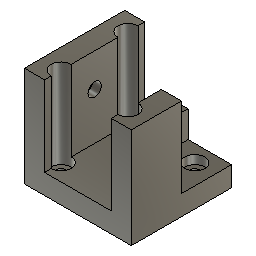
halter rakel neu v3 (Autodesk Fusion 360 design; units mm, degrees)
Autodesk Fusion 360 part; units mm, degrees
note: some values were not read from the file. Chosen so that the rebuilt part matches the saved one: which bodies a step acts on.
sketch "Skizze1" plane through (0, 0, 0) normal (0, 0, 1) x (1, 0, 0)
  line L0 (0, 0) -> (30, 0)
  line L1 (30, 0) -> (30, 30)
  line L2 (30, 30) -> (0, 30)
  line L3 (0, 30) -> (0, 0)
  line L4 (5, 25) -> (25, 25)
  line L5 (25, 25) -> (25, 5)
  line L6 (25, 5) -> (5, 5)
  line L7 (5, 5) -> (5, 25)
  circle A0 centre (5, 25) radius 1.5
  circle A1 centre (25, 25) radius 1.5
  circle A2 centre (5, 5) radius 1.5
  circle A3 centre (25, 5) radius 1.5
  dimension "d1" = 3
  dimension "d2" = 3
  dimension "d3" = 3
  dimension "d4" = 3
  constraint horizontal L0
  constraint vertical L1
  constraint horizontal L2
  constraint vertical L3
  constraint coincident L0.start L3.end
  constraint horizontal L4
  constraint vertical L5
  constraint horizontal L6
  constraint vertical L7
  constraint coincident L4.start L7.end
  constraint coincident L4.end L5.start
  constraint coincident L6.end L7.start
  constraint coincident L5.end L6.start
  measures "d1" diameter of A0
  measures "d2" diameter of A1
  measures "d3" diameter of A2
  measures "d4" diameter of A3
extrude "Extrusion1" add sketch "Skizze1" along normal blind 6 contours L0 L1 L2 L3 | L4 L5 L6 L7 A0 A1 A2 A3 makes body 1
sketch "Skizze2" plane through (0, 0, 6) normal (0, 0, 1) x (-1, 0, 0)
  circle A0 centre (-25, -5) radius 1.5
  circle A1 centre (-25, -25) radius 1.5
  circle A2 centre (-5, -5) radius 1.5
  circle A3 centre (-5, -25) radius 1.5
  line L0 (0, -30) -> (0, 0)
  line L1 (0, 0) -> (-30, 0)
  line L2 (-30, 0) -> (-30, -30)
  line L3 (-30, -30) -> (0, -30)
  circle A4 centre (-5, -25) radius 3
  circle A5 centre (-25, -25) radius 3
  circle A6 centre (-5, -5) radius 3
  circle A7 centre (-25, -5) radius 3
  dimension "d7" = 6
  dimension "d8" = 6
  dimension "d9" = 6
  dimension "d10" = 6
  constraint concentric A3 A4
  constraint concentric A1 A5
  constraint concentric A2 A6
  constraint concentric A0 A7
  measures "d7" diameter of A4
  measures "d8" diameter of A5
  measures "d9" diameter of A6
  measures "d10" diameter of A7
extrude "Extrusion2" cut sketch "Skizze2" against normal blind 2.6 contours A4 | A5 | A6 | A7 bodies 1
sketch "Skizze3" plane through (0, 0, 0) normal (0, 0, -1) x (1, 0, 0)
  circle A0 centre (25, -5) radius 1.5
  circle A1 centre (25, -25) radius 1.5
  circle A2 centre (5, -5) radius 1.5
  circle A3 centre (5, -25) radius 1.5
  line L0 (0, 0) -> (0, -30)
  line L1 (0, -30) -> (30, -30)
  line L2 (30, -30) -> (30, 0)
  line L3 (30, 0) -> (0, 0)
  line L4 (-5, 0) -> (35, 0)
  line L5 (35, 0) -> (35, -30)
  line L6 (35, -30) -> (-5, -30)
  line L7 (-5, -30) -> (-5, 0)
  constraint horizontal L4
  constraint vertical L5
  constraint horizontal L6
  constraint vertical L7
extrude "Extrusion3" add sketch "Skizze3" against normal blind 30 contours L0 L4 L6 L7 | L2 L4 L5 L6 bodies 1
extrude "Extrusion4" add 2 faces at (-3.3333, 10, 30) (31.6667, 10, 30) along direction (0, 0, 1) blind 10 on bodies 1 bodies 1
sketch "Skizze4" plane through (0, 0, 0) normal (1, 0, 0) x (0, 1, 0)
  line L0 (0, 6) -> (30, 6)
  line L1 (30, 6) -> (30, 40)
  line L2 (30, 40) -> (0, 40)
  line L3 (0, 40) -> (0, 6)
  line L4 (15, 40) -> (12, 40)
  line L5 (12, 40) -> (18, 40)
  line L6 (18, 40) -> (18, 5)
  line L7 (18, 5) -> (12, 5)
  line L8 (12, 5) -> (12, 40)
  dimension "d17" = 6
  dimension "d18" = 35
  constraint midpoint L2 L4.start
  constraint coincident L2 L4.end
  constraint perpendicular L1 L4
  constraint horizontal L5
  constraint vertical L6
  constraint horizontal L7
  constraint vertical L8
  measures "d17" distance of L4.end L5.end
  measures "d18" distance of L4.end L7.end
extrude "Extrusion5" add sketch "Skizze4" along normal blind 30 contours L0 L2 L4 L5 L6 L8 bodies 1
sketch "Skizze5" plane through (0, 0, 40) normal (0, 0, 1) x (-1, 0, 0)
  line L0 (0, -30) -> (5, -30)
  line L1 (5, -30) -> (5, 0)
  line L2 (5, 0) -> (0, 0)
  line L3 (0, 0) -> (0, -12)
  line L4 (0, -12) -> (-30, -12)
  line L5 (-30, -12) -> (-30, 0)
  line L6 (-30, 0) -> (-35, 0)
  line L7 (-35, 0) -> (-35, -30)
  line L8 (-35, -30) -> (-30, -30)
  line L9 (-30, -30) -> (-30, -18)
  line L10 (-30, -18) -> (0, -18)
  line L11 (0, -18) -> (0, -30)
  line L12 (0, -15) -> (-5, -15)
  line L13 (-30, -15) -> (-25, -15)
  line L14 (-5, -18) -> (-5, -12)
  line L15 (-5, -12) -> (-25, -12)
  line L16 (-25, -12) -> (-25, -18)
  line L17 (-25, -18) -> (-5, -18)
  constraint horizontal L12
  constraint parallel L12 L13
  constraint coincident L10 L14.start
  constraint coincident L4 L14.end
  constraint perpendicular L4 L14
  constraint coincident L4 L15.end
  constraint coincident L10 L16.end
  constraint perpendicular L10 L16
extrude "Extrusion6" cut sketch "Skizze5" against normal blind 34 contours L4 L10 L14 L15 L16 L17 bodies 1
extrude "Extrusion7" add 1 faces at (25, 14, 28.6667) along direction (-1, 0, 0) blind 5 on bodies 1 bodies 1
extrude "Extrusion8" add 1 faces at (5, 16, 28.6667) along direction (1, 0, 0) blind 5 on bodies 1 bodies 1
extrude "Extrusion9" add 2 faces at (30, 26, 17.3333) (30, 8, 17.3333) along direction (-1, 0, 0) blind 5 on bodies 1 bodies 1
extrude "Extrusion10" add 2 faces at (0, 4, 17.3333) (0, 22, 17.3333) along direction (1, 0, 0) blind 5 on bodies 1 bodies 1
extrude "Extrusion11" cut 4 faces at (2.5168, 5.2236, 3.4) (2.5168, 25.2236, 3.4) (22.5168, 25.2236, 3.4) (22.5168, 5.2236, 3.4) along direction (0, 0, 1) blind 46 on bodies 1 bodies 1 makes body 2 at (3.5561, 25.4063, 28.6667) makes body 3 at (25.1494, 3.5075, 28.6667) makes body 4 at (4.9252, 6.4981, 28.6667) makes body 5 at (26.4439, 24.5937, 28.6667)
extrude "Extrusion12" cut 2 faces at (25, 5.5, 28.6667) (25, 25.5, 17.3333) along direction (1, 0, 0) blind 2.5 on bodies 3 5 bodies 3 5
extrude "Extrusion13" cut 2 faces at (5, 25.5, 28.6667) (5, 5.5, 28.6667) along direction (-1, 0, 0) blind 2 on bodies 2 4 bodies 2 4
extrude "Extrusion14" cut 1 faces at (35, 10, 13.3333) along direction (-1, 0, 0) blind 4 on bodies 1 bodies 1
extrude "Extrusion15" cut 1 faces at (-5, 20, 13.3333) along direction (1, 0, 0) blind 4 on bodies 1 bodies 1
sketch "Skizze6" plane through (0, 12, 0) normal (0, -1, 0) x (1, 0, 0)
  line L0 (5, 40) -> (5, 6)
  line L1 (5, 6) -> (10, 6)
  line L2 (10, 6) -> (10, 40)
  line L3 (10, 40) -> (5, 40)
  line L4 (5, 35) -> (25, 35)
  line L5 (25, 35) -> (25, 11)
  line L6 (25, 11) -> (5, 11)
  line L7 (5, 11) -> (5, 35)
  constraint horizontal L4
  constraint vertical L5
  constraint horizontal L6
  constraint vertical L7
  constraint coincident L0 L4.start
extrude "Extrusion16" cut sketch "Skizze6" against normal blind 14 contours L0 L2 L4 L6 L7 | L2 L4 L5 L6 bodies 1
sketch "Skizze8" plane through (31, 0, 0) normal (1, 0, 0) x (0, 1, 0)
  circle A0 centre (15, 20) radius 2
  dimension "d48" = 4
  measures "d48" diameter of A0
extrude "Extrusion17" cut sketch "Skizze8" against normal blind 35 bodies 1
sketch "Skizze9" plane through (31, 0, 0) normal (1, 0, 0) x (0, 1, 0)
  circle A0 centre (15, 20) radius 2
  line L0 (0, 0) -> (30, 0)
  line L1 (30, 0) -> (30, 40)
  line L2 (30, 40) -> (0, 40)
  line L3 (0, 40) -> (0, 0)
  circle A1 centre (15, 20) radius 3.5
  dimension "d52" = 7
  constraint concentric A0 A1
  measures "d52" diameter of A1
extrude "Extrusion18" cut sketch "Skizze9" against normal blind 3.5 contours A1 bodies 1
sketch "Skizze10" plane through (-1, 0, 0) normal (-1, 0, 0) x (0, -1, 0)
  circle A0 centre (-15, 20) radius 2
  line L0 (-30, 0) -> (0, 0)
  line L1 (0, 0) -> (0, 40)
  line L2 (0, 40) -> (-30, 40)
  line L3 (-30, 40) -> (-30, 0)
  circle A1 centre (-15, 20) radius 3.5
  dimension "d55" = 7
  constraint concentric A0 A1
  measures "d55" diameter of A1
extrude "Extrusion19" cut sketch "Skizze10" against normal blind 3.5 contours A1 bodies 1
extrude "Extrusion20" add 2 faces at (6.6667, 14, 35) (21.6667, 14, 35) along direction (0, 0, -1) blind 6 on bodies 1 bodies 1 2 3 4 5
extrude "Extrusion21" cut 2 faces at (23.3333, 14, 11) (8.3333, 14, 11) along direction (0, 0, 1) blind 63 on bodies 1 bodies 1
extrude "Extrusion22" cut 2 faces at (8.3333, 14, 11) (23.3333, 14, 11) along direction (0, 0, -1) blind 5 on bodies 1 bodies 1
sketch "Skizze11" plane through (0, 0, 6) normal (0, 0, 1) x (-1, 0, 0)
  line L0 (-5, -22) -> (-5, -8)
  arc A0 (-5, -2) -> (-5, -8) centre (-5, -5) ccw
  line L1 (-5, -2) -> (-5, 0)
  line L2 (-5, 0) -> (-25, 0)
  line L3 (-25, 0) -> (-25, -2)
  arc A1 (-25, -8) -> (-25, -2) centre (-25, -5) ccw
  line L4 (-25, -8) -> (-25, -22)
  arc A2 (-25, -28) -> (-25, -22) centre (-25, -25) ccw
  line L5 (-25, -28) -> (-25, -30)
  line L6 (-25, -30) -> (-5, -30)
  line L7 (-5, -30) -> (-5, -28)
  arc A3 (-5, -22) -> (-5, -28) centre (-5, -25) ccw
  line L8 (-15, -30) -> (-12, -30)
  line L9 (-12, -30) -> (-18, -30)
  line L10 (-12, -30) -> (-12, -25)
  line L11 (-12, -25) -> (-18, -25)
  line L12 (-18, -25) -> (-18, -30)
  line L13 (-15, 0) -> (-12, 0)
  line L14 (-12, 0) -> (-12, -5)
  line L15 (-12, -5) -> (-18, -5)
  line L16 (-18, -5) -> (-18, 0)
  line L17 (-18, 0) -> (-15, 0)
  dimension "d64" = 3
  constraint midpoint L6 L8.start
  constraint parallel L6 L8
  constraint coincident L6 L9.end
  constraint perpendicular L9 L10
  constraint perpendicular L10 L11
  constraint perpendicular L6 L12
  constraint midpoint L2 L13.start
  constraint coincident L2 L13.end
  constraint perpendicular L12 L13
  constraint perpendicular L13 L14
  constraint perpendicular L14 L15
  constraint coincident L2 L16.end
  constraint perpendicular L2 L16
  measures "d64" distance of L8.start L8.end
extrude "Extrusion23" add sketch "Skizze11" along normal blind 8 contours L6 L8 L9 L10 L11 L12 | L2 L13 L14 L15 L16 L17 bodies 1
extrude "Extrusion24" cut 1 faces at (14, 5, 8.6667) along direction (0, -1, 0) blind 9 on bodies 1 bodies 1
extrude "Extrusion25" cut 2 faces at (29.9749, 11.8892, 40) (0.0405, 11.9484, 40) along direction (0, 0, -1) blind 10 on bodies 1 bodies 1
sketch "Skizze12" plane through (0, 0, 6) normal (0, 0, 1) x (-1, 0, 0)
  line L0 (-18, -30) -> (-18, -25)
  line L1 (-18, -25) -> (-12, -25)
  line L2 (-12, -25) -> (-12, -30)
  line L3 (-12, -30) -> (-5, -30)
  line L4 (-5, -30) -> (-5, -28)
  arc A0 (-5, -22) -> (-5, -28) centre (-5, -25) ccw
  line L5 (-5, -22) -> (-5, -8)
  arc A1 (-5, -2) -> (-5, -8) centre (-5, -5) ccw
  line L6 (-5, -2) -> (-5, 0)
  line L7 (-5, 0) -> (-25, 0)
  line L8 (-25, 0) -> (-25, -2)
  arc A2 (-25, -8) -> (-25, -2) centre (-25, -5) ccw
  line L9 (-25, -8) -> (-25, -22)
  arc A3 (-25, -28) -> (-25, -22) centre (-25, -25) ccw
  line L10 (-25, -28) -> (-25, -30)
  line L11 (-25, -30) -> (-18, -30)
  line L12 (-25, -5) -> (-5, -5)
  line L13 (-5, -5) -> (-5, -25)
  line L14 (-5, -25) -> (-25, -25)
  line L15 (-25, -25) -> (-25, -5)
  line L16 (-18, -25) -> (-12, -25)
  line L17 (-12, -25) -> (-12, -20)
  line L18 (-12, -20) -> (-18, -20)
  line L19 (-18, -20) -> (-18, -25)
  dimension "d71" = 5
  constraint horizontal L12
  constraint vertical L13
  constraint horizontal L14
  constraint vertical L15
  constraint coincident A0.centre L13.end
  constraint coincident A2.centre L12.start
  constraint horizontal L16
  constraint vertical L17
  constraint horizontal L18
  constraint vertical L19
  constraint coincident L0.end L1.start
  measures "d71" distance of L0.end L18.end
extrude "Extrusion26" add sketch "Skizze12" along normal blind 8 contours L1 L14 L16 L17 L18 L19 bodies 1
sketch "Skizze13" plane through (0, 0, 30) normal (0, 0, 1) x (-1, 0, 0)
  line L0 (-25, -22) -> (-25, -8)
  arc A0 (-25, -2) -> (-25, -8) centre (-25, -5) ccw
  line L1 (-25, -2) -> (-25, 0)
  line L2 (-25, 0) -> (-31, 0)
  line L3 (-31, 0) -> (-31, -30)
  line L4 (-31, -30) -> (-25, -30)
  line L5 (-25, -30) -> (-25, -28)
  arc A1 (-25, -22) -> (-25, -28) centre (-25, -25) ccw
  line L6 (-31, 0) -> (-25, 0)
  line L7 (-25, 0) -> (-25, -15)
  line L8 (-25, -15) -> (-31, -15)
  line L9 (-31, -15) -> (-31, 0)
  constraint horizontal L6
  constraint vertical L7
  constraint horizontal L8
  constraint vertical L9
  constraint midpoint L0 L7.end
  constraint coincident L2.end L3.start
extrude "Extrusion29" cut sketch "Skizze13" against normal blind 24 contours L0 L3 L4 L5 A1 L8 bodies 1
sketch "Skizze15" plane through (31, 0, 0) normal (1, 0, 0) x (0, 1, 0)
  line L0 (30, 6) -> (15, 6)
  line L1 (15, 6) -> (15, 16.5)
  arc A0 (15, 23.5) -> (15, 16.5) centre (15, 20) ccw
  line L2 (15, 23.5) -> (15, 30)
  line L3 (15, 30) -> (0, 30)
  line L4 (0, 30) -> (0, 0)
  line L5 (0, 0) -> (30, 0)
  line L6 (30, 0) -> (30, 6)
  line L7 (15, 25) -> (11, 25)
  line L8 (11, 25) -> (11, 15)
  line L9 (11, 15) -> (15, 15)
  line L10 (15, 15) -> (15, 25)
  constraint horizontal L7
  constraint vertical L8
  constraint horizontal L9
  constraint vertical L10
  constraint coincident L2 L7.start
extrude "Extrusion30" add sketch "Skizze15" against normal blind 6 contours A0 L10 bodies 1
